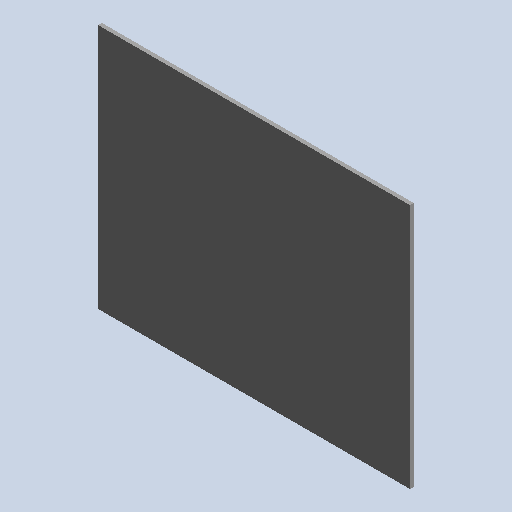
# Autodesk Inventor part: layer1
Saved by Autodesk Inventor 2026 (Build 300175050, 175E)
## iProperties
Part Number: layer1
Material: Generic
Document SubType Name: Modeling
Designer: Kartik
Mass: 343.2 g
Surface Area: 1763.2 cm^2
Volume: 343.2 cm^3
Density: 1 g/cm^3
Appearance: Default
Author: Kartik
Autodesk Inventor part; units mm, degrees
ref_plane "YZ Plane" through (0, 0, 0) normal (1, 0, 0) x (0, 1, 0)
ref_plane "XZ Plane" through (0, 0, 0) normal (0, 1, 0) x (-1, 0, 0)
ref_plane "XY Plane" through (0, 0, 0) normal (0, 0, 1) x (1, 0, 0)
sketch "Sketch1" plane through (0, 0, 0) normal (0, 0, 1) x (1, 0, 0)
  line L0 (-186.75, 109.875) -> (143.25, 109.875)
  line L1 (143.25, 109.875) -> (143.25, -150.125)
  line L2 (143.25, -150.125) -> (-186.75, -150.125)
  line L3 (-186.75, -150.125) -> (-186.75, 109.875)
  point P0 (0, 0)
  dimension "d0" = 330
  dimension "d1" = 260
  constraints: 8 end point, 2 parallel, 1 horizontal, 1 perpendicular
  measures "d0" distance of L0.start L0.end
  measures "d1" distance of L0.end L1.end
extrude "Extrusion1" add sketch "Sketch1" along normal blind 4
body "Solid1"
